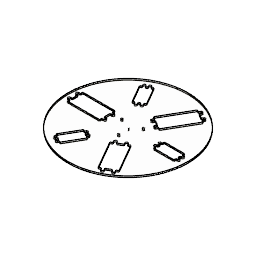
BaseV0_v17 (Autodesk Fusion 360 design; units mm, degrees)
Autodesk Fusion 360 part; units mm, degrees
sketch "Sketch1" plane through (0, 0, 0) normal (0, 0, 1) x (1, 0, 0)
  circle A0 centre (0, 0) radius 125
  line L0 (0, 0) -> (125, 0) construction
  line L1 (107, -11) -> (65, -11)
  line L2 (65, -11) -> (65, 11)
  line L3 (65, 11) -> (107, 11)
  line L4 (107, 11) -> (107, -11)
  line L5 (107, -11) -> (65, 11) construction
  line L6 (65, -11) -> (107, 11) construction
  line L7 (61.76, 0) -> (110.24, 0) construction
  line L8 (110.24, 4.5) -> (110.24, -4.5) construction
  line L9 (61.76, 4.5) -> (61.76, -4.5) construction
  circle A1 centre (110.24, 4.5) radius 2.5
  circle A2 centre (110.24, -4.5) radius 2.5
  circle A3 centre (61.76, 4.5) radius 2.5
  circle A4 centre (61.76, -4.5) radius 2.5
  line L10 (61.76, 4.5) -> (61.76, 7) construction
  line L11 (61.76, 7) -> (65, 7)
  line L12 (61.76, 4.5) -> (61.76, 2) construction
  line L13 (61.76, 2) -> (65, 2)
  line L14 (61.76, -4.5) -> (61.76, -2) construction
  line L15 (61.76, -4.5) -> (61.76, -7) construction
  line L16 (61.76, -2) -> (65, -2)
  line L17 (61.76, -7) -> (65, -7)
  line L18 (110.24, 4.5) -> (110.24, 7) construction
  line L19 (110.24, 7) -> (107, 7)
  line L20 (110.24, 2) -> (107, 2)
  line L21 (110.24, -2) -> (107, -2)
  line L22 (110.24, -7) -> (107, -7)
  line L23 (-26.9829, 55.7357) -> (-29.1479, 54.4857) construction
  line L24 (-43.9737, 98.1647) -> (-42.0263, 50.7917) construction
  circle A5 centre (-34.7771, 51.2357) radius 2.5
  line L25 (-26.9829, 55.7357) -> (-24.8178, 56.9857) construction
  line L26 (-43.9737, 98.1647) -> (-22.9737, 61.7917)
  line L27 (-30.88, 53.4857) -> (-55.12, 95.4706) construction
  line L28 (-22.9737, 61.7917) -> (-63.0263, 87.1647) construction
  line L29 (-29.1479, 54.4857) -> (-30.7679, 57.2917)
  line L30 (-56.8521, 94.4706) -> (-55.2321, 91.6647)
  line L31 (-49.0578, 98.9706) -> (-47.4378, 96.1647)
  line L32 (-53.3879, 96.4706) -> (-51.7679, 93.6647)
  line L33 (-59.0171, 93.2206) -> (-61.1822, 91.9706) construction
  line L34 (-22.9737, 61.7917) -> (-42.0263, 50.7917)
  circle A6 centre (-51.2229, 97.7206) radius 2.5
  line L35 (-61.1822, 91.9706) -> (-59.5622, 89.1647)
  line L36 (-24.8178, 56.9857) -> (-26.4378, 59.7917)
  line L37 (-63.0263, 87.1647) -> (-43.9737, 98.1647)
  line L38 (-32.6121, 52.4857) -> (-34.2321, 55.2917)
  line L39 (-34.7771, 51.2357) -> (-32.6121, 52.4857) construction
  line L40 (-34.7771, 51.2357) -> (-26.9829, 55.7357) construction
  line L41 (-34.7771, 51.2357) -> (-36.9422, 49.9857) construction
  line L42 (-42.0263, 50.7917) -> (-63.0263, 87.1647)
  circle A7 centre (-26.9829, 55.7357) radius 2.5
  line L43 (-59.0171, 93.2206) -> (-51.2229, 97.7206) construction
  circle A8 centre (-59.0171, 93.2206) radius 2.5
  line L44 (-36.9422, 49.9857) -> (-38.5622, 52.7917)
  line L45 (-34.7771, -51.2357) -> (-32.6121, -52.4857) construction
  line L46 (-63.0263, -87.1647) -> (-22.9737, -61.7917) construction
  circle A9 centre (-26.9829, -55.7357) radius 2.5
  line L47 (-34.7771, -51.2357) -> (-36.9422, -49.9857) construction
  line L48 (-63.0263, -87.1647) -> (-42.0263, -50.7917)
  line L49 (-30.88, -53.4857) -> (-55.12, -95.4706) construction
  line L50 (-42.0263, -50.7917) -> (-43.9737, -98.1647) construction
  line L51 (-32.6121, -52.4857) -> (-34.2321, -55.2917)
  line L52 (-53.3879, -96.4706) -> (-51.7679, -93.6647)
  line L53 (-61.1822, -91.9706) -> (-59.5622, -89.1647)
  line L54 (-56.8521, -94.4706) -> (-55.2321, -91.6647)
  line L55 (-51.2229, -97.7206) -> (-49.0578, -98.9706) construction
  line L56 (-42.0263, -50.7917) -> (-22.9737, -61.7917)
  circle A10 centre (-59.0171, -93.2206) radius 2.5
  line L57 (-49.0578, -98.9706) -> (-47.4378, -96.1647)
  line L58 (-36.9422, -49.9857) -> (-38.5622, -52.7917)
  line L59 (-43.9737, -98.1647) -> (-63.0263, -87.1647)
  line L60 (-29.1479, -54.4857) -> (-30.7679, -57.2917)
  line L61 (-26.9829, -55.7357) -> (-29.1479, -54.4857) construction
  line L62 (-26.9829, -55.7357) -> (-34.7771, -51.2357) construction
  line L63 (-26.9829, -55.7357) -> (-24.8178, -56.9857) construction
  line L64 (-22.9737, -61.7917) -> (-43.9737, -98.1647)
  circle A11 centre (-34.7771, -51.2357) radius 2.5
  line L65 (-51.2229, -97.7206) -> (-59.0171, -93.2206) construction
  circle A12 centre (-51.2229, -97.7206) radius 2.5
  line L66 (-24.8178, -56.9857) -> (-26.4378, -59.7917)
  circle A13 centre (3.1919, -22.7115) radius 2.1
  circle A14 centre (-21.2647, 8.5915) radius 2.1
  circle A15 centre (18.0728, 14.12) radius 2.1
  line L67 (0, 0) -> (62.5, 108.2532) construction
  line L68 (0, 0) -> (-62.5, 108.2532) construction
  line L69 (0, 0) -> (-125, 0) construction
  line L70 (0, 0) -> (-62.5, -108.2532) construction
  line L71 (0, 0) -> (62.5, -108.2532) construction
  line L72 (-43.5879, -16) -> (-110.5879, -16)
  line L73 (-110.5879, -16) -> (-110.5879, 16)
  line L74 (-110.5879, 16) -> (-43.5879, 16)
  line L75 (-43.5879, 16) -> (-43.5879, -16)
  line L76 (-43.5879, -16) -> (-110.5879, 16) construction
  line L77 (-110.5879, -16) -> (-43.5879, 16) construction
  line L78 (-39.5879, -8.5) -> (-114.5879, -8.5) construction
  line L79 (-114.5879, -8.5) -> (-114.5879, 8.5) construction
  line L80 (-114.5879, 8.5) -> (-39.5879, 8.5) construction
  line L81 (-39.5879, 8.5) -> (-39.5879, -8.5) construction
  line L82 (-39.5879, -8.5) -> (-114.5879, 8.5) construction
  line L83 (-114.5879, -8.5) -> (-39.5879, 8.5) construction
  circle A16 centre (-114.5879, 8.5) radius 2.65
  circle A17 centre (-114.5879, -8.5) radius 2.65
  line L84 (-114.5879, 8.5) -> (-114.5879, 11.15) construction
  line L85 (-114.5879, 11.15) -> (-110.5879, 11.15)
  line L86 (-114.5879, 8.5) -> (-114.5879, 5.85) construction
  line L87 (-114.5879, 5.85) -> (-110.5879, 5.85)
  line L88 (-114.5879, -8.5) -> (-114.5879, -5.85) construction
  line L89 (-114.5879, -5.85) -> (-110.5879, -5.85)
  line L90 (-114.5879, -8.5) -> (-114.5879, -11.15) construction
  line L91 (-114.5879, -11.15) -> (-110.5879, -11.15)
  line L92 (-77.0879, 0) -> (-77.0879, 3.2461) construction
  line L93 (-39.5879, 11.15) -> (-43.5879, 11.15)
  circle A18 centre (-39.5879, 8.5) radius 2.65
  line L94 (-39.5879, 5.85) -> (-43.5879, 5.85)
  line L95 (-39.5879, -5.85) -> (-43.5879, -5.85)
  circle A19 centre (-39.5879, -8.5) radius 2.65
  line L96 (-39.5879, -11.15) -> (-43.5879, -11.15)
  line L97 (-77.0879, 0) -> (-77.0879, 3.2461) construction
  line L98 (41.4375, -103.7719) -> (7.9375, -45.7482)
  line L99 (69.1503, -87.7719) -> (41.4375, -103.7719)
  line L100 (47.6377, -104.811) -> (45.6377, -101.3469)
  circle A20 centre (49.9327, -103.486) radius 2.65
  line L101 (52.2277, -102.161) -> (50.2277, -98.6969)
  line L102 (62.3602, -96.311) -> (60.3602, -92.8469)
  line L103 (35.6503, -29.7482) -> (69.1503, -87.7719)
  line L104 (66.9501, -93.661) -> (64.9501, -90.1969)
  circle A21 centre (64.6551, -94.986) radius 2.65
  circle A22 centre (12.4327, -38.5341) radius 2.65
  line L105 (10.1377, -39.8591) -> (12.1377, -43.3232)
  line L106 (7.9375, -45.7482) -> (35.6503, -29.7482)
  line L107 (14.7277, -37.2091) -> (16.7277, -40.6732)
  line L108 (24.8602, -31.3591) -> (26.8602, -34.8232)
  circle A23 centre (27.1551, -30.0341) radius 2.65
  line L109 (29.4501, -28.7091) -> (31.4501, -32.1732)
  line L110 (69.1503, 87.7719) -> (35.6503, 29.7482)
  line L111 (41.4375, 103.7719) -> (69.1503, 87.7719)
  line L112 (66.9501, 93.661) -> (64.9501, 90.1969)
  circle A24 centre (64.6551, 94.986) radius 2.65
  line L113 (62.3602, 96.311) -> (60.3602, 92.8469)
  line L114 (52.2277, 102.161) -> (50.2277, 98.6969)
  line L115 (7.9375, 45.7482) -> (41.4375, 103.7719)
  line L116 (47.6377, 104.811) -> (45.6377, 101.3469)
  circle A25 centre (49.9327, 103.486) radius 2.65
  circle A26 centre (27.1551, 30.0341) radius 2.65
  line L117 (29.4501, 28.7091) -> (31.4501, 32.1732)
  line L118 (35.6503, 29.7482) -> (7.9375, 45.7482)
  line L119 (24.8602, 31.3591) -> (26.8602, 34.8232)
  line L120 (14.7277, 37.2091) -> (16.7277, 40.6732)
  circle A27 centre (12.4327, 38.5341) radius 2.65
  line L121 (10.1377, 39.8591) -> (12.1377, 43.3232)
  circle A28 centre (3.1787, -1.7716) radius 1
  circle A29 centre (0, 0) radius 2
  line L122 (3.1787, -1.7716) -> (0, 0)
  point P0 (0, 0)
  point P1 (86, 0)
  point P2 (86, 0)
  point P3 (-43, 74.4782)
  point P4 (-43, 74.4782)
  point P5 (-43, -74.4782)
  point P6 (-43, -74.4782)
  point P7 (-77.0879, 0)
  point P8 (-77.0879, 0)
  dimension "d7" = 250
  dimension "d12" = 42
  dimension "d13" = 22
  dimension "d14" = 65
  dimension "d15" = 48.48
  dimension "d16" = 9
  dimension "d17" = 9
  dimension "d18" = 5
  dimension "d19" = 5
  dimension "d20" = 5
  dimension "d21" = 5
  dimension "d23" = 360
  dimension "d28" = 4.2
  dimension "d30" = 360
  dimension "d31" = 32
  dimension "d32" = 67
  dimension "d33" = 75
  dimension "d34" = 17
  dimension "d35" = 5.3
  dimension "d36" = 5.3
  dimension "d38" = 360
  constraint coincident A0.centre L0.start
  constraint coincident P0 A0.centre
  constraint coincident A0 L0.end
  constraint horizontal L1
  constraint perpendicular L1 L2
  constraint parallel L1 L3
  constraint parallel L2 L4
  constraint coincident L5 P2
  constraint coincident L6 P2
  constraint coincident L0 P2
  constraint coincident L0 P0
  constraint midpoint L7 P2
  constraint coincident P2 P1
  constraint perpendicular L4 L7
  constraint midpoint L7.end L8
  constraint perpendicular L0 L8
  constraint midpoint L7.start L9
  constraint perpendicular L0 L9
  constraint coincident L8.start A1.centre
  constraint coincident L8.end A2.centre
  constraint coincident L9.start A3.centre
  constraint coincident L9.end A4.centre
  constraint coincident A3 L10.end
  constraint vertical L10
  constraint coincident L2 L11.end
  constraint perpendicular L2 L11
  constraint coincident A3 L12.end
  constraint coincident L9 L12.end
  constraint coincident L2 L13.end
  constraint perpendicular L2 L13
  constraint coincident A4 L14.end
  constraint coincident L9 L14.end
  constraint coincident A4 L15.end
  constraint parallel L9 L15
  constraint coincident L2 L16.end
  constraint perpendicular L2 L16
  constraint coincident L2 L17.end
  constraint perpendicular L2 L17
  constraint coincident A1 L18.end
  constraint parallel L8 L18
  constraint coincident L4 L19.end
  constraint perpendicular L4 L19
  constraint coincident L8 L20.start
  constraint coincident A1 L20.start
  constraint coincident L4 L20.end
  constraint tangent A1 L20
  constraint coincident A2 L21.start
  constraint coincident L8 L21.start
  constraint coincident L4 L21.end
  constraint tangent A2 L21
  constraint coincident A2 L22.start
  constraint coincident L4 L22.end
  constraint tangent A2 L22
  constraint perpendicular L4 L22
  constraint horizontal L72
  constraint perpendicular L72 L73
  constraint parallel L72 L74
  constraint parallel L73 L75
  constraint coincident L76 P8
  constraint coincident L77 P8
  constraint coincident L69 P8
  constraint horizontal L78
  constraint perpendicular L78 L79
  constraint parallel L78 L80
  constraint parallel L79 L81
  constraint coincident L82 P8
  constraint coincident L83 P8
  constraint coincident P8 P7
  constraint coincident L79.end L80.start
  constraint coincident L78.end L79.start
  constraint coincident A16 L84.end
  constraint perpendicular L80 L84
  constraint coincident L73 L85.end
  constraint tangent A16 L85
  constraint coincident A16 L86.end
  constraint coincident L79 L86.end
  constraint coincident L73 L87.end
  constraint tangent A16 L87
  constraint coincident A17 L88.end
  constraint coincident L79 L88.end
  constraint coincident L73 L89.end
  constraint tangent A17 L89
  constraint coincident A17 L90.end
  constraint perpendicular L78 L90
  constraint coincident L73 L91.end
  constraint tangent A17 L91
  constraint symmetric A16 L92 A18
  constraint symmetric A17 L92 A19
  constraint symmetric L84.end L92 L93.start
  constraint symmetric L85.end L92 L93.end
  constraint symmetric L86.end L92 L94.start
  constraint symmetric L87.end L92 L94.end
  constraint symmetric L88.end L92 L95.start
  constraint symmetric L89.end L92 L95.end
  constraint symmetric L90.end L92 L96.start
  constraint symmetric L91.end L92 L96.end
  constraint symmetric P8 L92 P7
  constraint symmetric L97.end L92 L92.end
  constraint coincident A28.centre L122.start
  measures "d7" diameter of A0
  measures "d12" distance of L2.end L3.end
  measures "d13" distance of L1.end L2.end
  measures "d14" distance of P0 L2
  measures "d15" distance of L7.start L7.end
  measures "d16" distance of L8.start L8.end
  measures "d17" distance of L9.start L9.end
  measures "d18" diameter of A1
  measures "d19" diameter of A2
  measures "d20" diameter of A3
  measures "d21" diameter of A4
  measures "d28" diameter of A13
  measures "d31" distance of L72.start L74.end
  measures "d32" distance of L73.end L74.end
  measures "d33" distance of L79.end L80.end
  measures "d34" distance of L78.end L79.end
  measures "d35" diameter of A16
  measures "d36" diameter of A17
extrude "Extrude4" add sketch "Sketch1" along normal blind 3 contours A0 | A29
equation "d36 = 2.65 * 2 mm"
